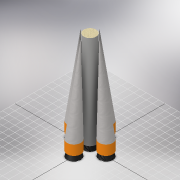
# Autodesk Inventor part: soyuz
Saved by Autodesk Inventor 2019 (Build 230136000, 136)
## iProperties
Created: 2020-11-05
Part Number: soyuz
Material: Generic
Document SubType Name: Modeling
Designer: Manoj
Density: 1 g/cm^3
Appearance: Diamond plate 2 - Dark Gray
Author: Manoj
Autodesk Inventor part; units mm, degrees
sketch "Sketch1" plane through (0, 0, 0) normal (0, 1, 0) x (-1, 0, 0)
  circle A0 centre (0, 0) radius 25
  dimension "d0" = 50
  constraints: 1 centre point, 1 coincident
  measures "d0" diameter of A0
ref_plane "Work Plane1" through (0, 50, 0) normal (0, 1, 0) x (-1, 0, 0)
sketch "Sketch2" plane through (0, 50, 0) normal (0, 1, 0) x (-1, 0, 0)
  circle A0 centre (0, 0) radius 11.5
  dimension "d2" = 23
  constraints: 1 centre point, 1 coincident
  measures "d2" diameter of A0
loft "Loft2" add profiles "Sketch1", "Sketch2"
ref_plane "Work Plane2" through (0, 20, 0) normal (0, -1, 0) x (1, 0, 0)
sketch "Sketch5" plane through (0, 20, 0) normal (0, -1, 0) x (1, 0, 0)
  circle A0 centre (0, 0) radius 25
  constraints: 1 centre point, 1 coincident
extrude "Extrusion1" add sketch "Sketch5" against normal blind 380
sketch "Sketch6" plane through (0, 0, 0) normal (0, 1, 0) x (-1, 0, 0)
  line L0 (0, 0) -> (0, 65)
  line L1 (0, 65) -> (0, -65)
  circle A0 centre (0, 65) radius 27.5
  dimension "d27" = 65
  dimension "d28" = 130
  dimension "d29" = 55
  constraints: 4 end point, 1 centre point, 1 coincident, 1 point on line, 1 vertical
  measures "d27" distance of L0.start L0.end
  measures "d28" distance of L0.end L1.end
  measures "d29" diameter of A0
ref_plane "Work Plane3" through (0, 50, 0) normal (0, 1, 0) x (-1, 0, 0)
sketch "Sketch7" plane through (0, 50, 0) normal (0, 1, 0) x (-1, 0, 0)
  circle A0 centre (0, 65) radius 14
  point P0 (0, 0)
  dimension "d32" = 28
  constraints: 1 centre point, 1 coincident
  measures "d32" diameter of A0
loft "Loft3" add profiles "Sketch6", "Sketch7"
ref_plane "Work Plane4" through (0, 20, 0) normal (0, 1, 0) x (-1, 0, 0)
pattern_circular "Circular Pattern1" count 4 over 360 about axis through (0, -10, 0) along (0, 1, 0) of "Loft3"
sketch "Sketch8" plane through (0, 20, 0) normal (0, 1, 0) x (-1, 0, 0)
  point P0 (0, 0)
sketch "Sketch9" plane through (0, 20, 0) normal (0, 1, 0) x (-1, 0, 0)
  line L0 (0, 0) -> (0, 65)
  circle A0 centre (0, 65) radius 27.5
  dimension "d41" = 65
  dimension "d42" = 55
  constraints: 2 end point, 1 centre point, 1 coincident, 1 vertical
  measures "d41" distance of L0.start L0.end
  measures "d42" diameter of A0
extrude "Extrusion2" add sketch "Sketch9" along normal blind 20
sketch "Sketch10" plane through (0, 40, 65) normal (0, 1, 0) x (1, 0, 0)
  line L0 (0, 65) -> (0, 0)
  circle A0 centre (0, 0) radius 27.5
  dimension "d45" = 65
  dimension "d46" = 55
  constraints: 2 end point, 1 centre point, 1 coincident, 1 vertical
  measures "d45" distance of L0.start L0.end
  measures "d46" diameter of A0
extrude "Extrusion3" add sketch "Sketch10" along normal blind 20
sketch "Sketch11" plane through (0, 400, 0) normal (0, 1, 0) x (1, 0, 0)
  circle A0 centre (0, -65) radius 27.5 projected
  circle A1 centre (0, -65) radius 27.5 projected
  point P0 (0, 0)
  point P1 (0, -37.5)
  constraints: 1 vertical alignment, 1 other
pattern_circular "Circular Pattern2" count 4 over 360 about axis through (0, -10, 0) along (0, 1, 0) of "Extrusion2", "Extrusion3"
loft "Loft4" add section 1 edges at (-27.5, 60, 65) section 2 point at (0, 400, 37.5)
pattern_circular "Circular Pattern3" count 4 over 360 about axis through (0, -10, 0) along (0, 1, 0) of "Loft4"
body "Solid2"
